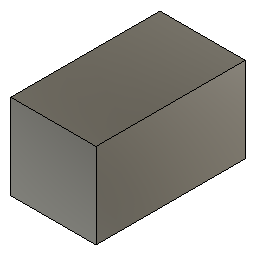
APIExample v5 (Autodesk Fusion 360 design; units mm, degrees)
Autodesk Fusion 360 part; units mm, degrees
sketch "Sketch1" plane through (0, 0, 0) normal (0, 0, 1) x (1, 0, 0)
  line L0 (508, 889) -> (-508, 889)
  line L1 (-508, 889) -> (-508, -889)
  line L2 (-508, -889) -> (508, -889)
  line L3 (508, -889) -> (508, 889)
  line L4 (508, 889) -> (-508, -889) construction
  line L5 (-508, 889) -> (508, -889) construction
  dimension "LengthValue" = 1778
  dimension "WidthValue" = 1016
  constraint horizontal L0
  constraint perpendicular L0 L1
  constraint parallel L0 L2
  constraint parallel L1 L3
  constraint coincident L4 origin
  constraint coincident L5 origin
  measures "LengthValue" distance of L0 L2
  measures "WidthValue" distance of L1 L3
extrude "Extrude1" add sketch "Sketch1" along normal blind 1016
equation "LengthValue = Length"
equation "WidthValue = Width"
equation "Heightvalue = Height"
equation "Height = 40 in"
equation "Width = 40 in"
equation "Length = 70 in"
